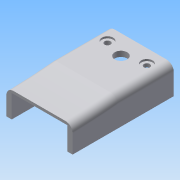
# Autodesk Inventor part: part1_top
Saved by Autodesk Inventor 2015 (Build 190159000, 159)
## iProperties
Created: 2015-08-21
Part Number: part1_top
Material: Générique
Document SubType Name: Modeling
Designer: Gregwar
Density: 1 g/cm^3
Appearance: Par défaut
Author: Gregwar
Autodesk Inventor part; units mm, degrees
ref_plane "YZ Plane" through (0, 0, 0) normal (1, 0, 0) x (0, 1, 0)
ref_plane "XZ Plane" through (0, 0, 0) normal (0, 1, 0) x (-1, 0, 0)
ref_plane "XY Plane" through (0, 0, 0) normal (0, 0, 1) x (1, 0, 0)
sketch "Esquisse1" plane through (0, 0, 0) normal (0, 1, 0) x (-1, 0, 0)
  line L0 (0, 0) -> (37, 0)
  line L1 (37, 0) -> (37, -31.5)
  line L2 (37, -31.5) -> (0, -31.5)
  line L3 (0, -31.5) -> (0, 0)
  line L4 (34, -28.5) -> (34, -3)
  line L5 (34, -3) -> (3, -3)
  line L6 (3, -3) -> (3, -28.5)
  line L7 (3, -28.5) -> (34, -28.5)
  line L8 (3, -15.75) -> (0, -15.75)
  line L9 (34, -15.75) -> (37, -15.75)
  dimension "d0" = 3
  dimension "d1" = 31
  dimension "d2" = 25.5
  constraints: 20 end point, 4 midpoint, 4 parallel, 2 perpendicular, 1 horizontal, 3 other
  measures "d0" distance between parallel lines of L7 L2
  measures "d1" distance of L4.end L5.end
  measures "d2" distance of L5.end L6.end
extrude "Extrusion1" add sketch "Esquisse1" along normal blind 56.5 contours L0 L1 L9 L4 L5 L6 L8 L3
sketch "Esquisse2" plane through (-37, 0, 0) normal (0, 0, 1) x (1, 0, 0)
  line L0 (7.5, 49) -> (29.5, 49) construction
  circle A0 centre (7.5, 49) radius 1.65
  circle A1 centre (29.5, 49) radius 1.65
  line L1 (34, 0) -> (3, 0) construction
  line L2 (18.5, 0) -> (18.5, 49) construction
  point P0 (37, 0)
  dimension "d5" = 3.3
  dimension "d6" = 49
  dimension "d7" = 22
  constraints: 4 end point, 2 centre point, 2 coincident, 2 midpoint, 1 equal radius, 1 perpendicular, 1 vertical
  measures "d5" diameter of A1
  measures "d6" distance of L2.start L2.end
  measures "d7" distance of A0.centre A1.centre
extrude "Extrusion2" cut sketch "Esquisse2" against normal through all
sketch "Esquisse3" plane through (-33, 0, 0) normal (0, 0, 1) x (1, 0, 0)
  line L0 (-4, 56.5) -> (33, 56.5) construction
  line L1 (-4, 0) -> (33, 0) construction
  circle A0 centre (3.5, 49) radius 1.65 construction
  circle A1 centre (25.5, 49) radius 1.65 construction
  circle A2 centre (3.5, 49) radius 1.65 construction
  circle A3 centre (3.5, 49) radius 3.15
  circle A4 centre (25.5, 49) radius 3.15
  line L2 (33, 0) -> (33, 56.5) projected
  line L3 (-4, 0) -> (-4, 56.5) projected
  dimension "d11" = 6.3
  constraints: 2 centre point, 2 coincident, 1 equal radius
  measures "d11" diameter of A4
extrude "Extrusion3" cut sketch "Esquisse3" against normal blind 1
sketch "Esquisse4" plane through (-33, 0, 0) normal (0, 0, 1) x (1, 0, 0)
  line L0 (-4, 56.5) -> (33, 56.5) construction
  line L1 (14.5, 56.5) -> (14.5, 0) construction
  line L2 (30, 0) -> (-1, 0) construction
  circle A0 centre (14.5, 45.5) radius 3.5
  point P0 (33, 0)
  point P1 (0, 56.5)
  point P2 (29, 56.5)
  dimension "d14" = 45.5
  dimension "d15" = 7
  constraints: 2 end point, 2 midpoint, 1 centre point, 1 point on line
  measures "d14" distance from line of L2 A0.centre
  measures "d15" diameter of A0
extrude "Extrusion4" cut sketch "Esquisse4" against normal through all
sketch "Esquisse5" plane through (0, 0, 0) normal (1, 0, 0) x (0, 0, -1)
  line L0 (0, 0) -> (1.5, 0)
  line L1 (0, 0) -> (15.75, 0) projected
  line L2 (0, 0) -> (0, 56.5) projected
  spline S0 degree 2 poles (1.5, 0) (1.2491, 12.5149) (0, 25) knots 0 0 0 1 1 1
  line L3 (0, 25) -> (0, 0)
  point P0 (1, 12.5)
  dimension "d18" = 1.5
  dimension "d19" = 25
  dimension "d20" = 12.5
  dimension "d21" = 1
  constraints: 4 end point, 2 point on line, 1 collinear, 3 other
  measures "d18" distance of L0.start L0.end
  measures "d19" distance of L0.start L3.start
  measures "d20" vertical distance of L0.start point (1, 12.5)
  measures "d21" distance from line of L2 point (1, 12.5)
extrude "Extrusion5" cut sketch "Esquisse5" against normal through all
fillet "Congé2" radius 4 4 edges at (0, 12.5075, -0.9996) (0, 40.75, 0) (-37, 40.75, 0) (-37, 12.5149, -0.9991)
fillet "Congé3" radius 1 3 edges at (-18.5, 25, 0) (-1.1716, 25, -1.1716) (-35.8284, 25, -1.1716)
equation "\"d20\" = 0.5 * d19"
